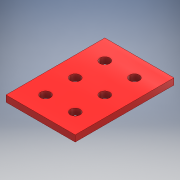
# Autodesk Inventor part: soportes celda de carga
Saved by Autodesk Inventor 2018 (Build 220112000, 112)
## iProperties
Created: 2019-05-18
Part Number: soportes celda de carga
Material: Generic
Document SubType Name: Modeling
Designer: JLVega003
Density: 1 g/cm^3
Appearance: Light Red
Author: JLVega003
Autodesk Inventor part; units mm, degrees
ref_plane "YZ Plane" through (0, 0, 0) normal (1, 0, 0) x (0, 1, 0)
ref_plane "XZ Plane" through (0, 0, 0) normal (0, 1, 0) x (-1, 0, 0)
ref_plane "XY Plane" through (0, 0, 0) normal (0, 0, 1) x (1, 0, 0)
sketch "Sketch1" plane through (0, 0, 0) normal (0, 0, 1) x (1, 0, 0)
  line L0 (17.5, -25) -> (-17.5, -25)
  line L1 (-17.5, -25) -> (-17.5, 25)
  line L2 (-17.5, 25) -> (17.5, 25)
  line L3 (17.5, 25) -> (17.5, -25)
  line L4 (17.5, -25) -> (-17.5, 25) construction
  line L5 (-17.5, -25) -> (17.5, 25) construction
  line L6 (7.5, -15) -> (-7.5, -15) construction
  line L7 (-7.5, -15) -> (-7.5, 15) construction
  line L8 (-7.5, 15) -> (7.5, 15) construction
  line L9 (7.5, 15) -> (7.5, -15) construction
  line L10 (7.5, -15) -> (-7.5, 15) construction
  line L11 (-7.5, -15) -> (7.5, 15) construction
  circle A0 centre (-7.5, 15) radius 2.5
  circle A1 centre (7.5, 15) radius 2.5
  circle A2 centre (-7.5, -15) radius 2.5
  circle A3 centre (7.5, -15) radius 2.5
  circle A4 centre (-7.5, 0) radius 2.5
  circle A5 centre (7.5, 0) radius 2.5
  point P0 (0, 0)
  dimension "d3" = 10
  dimension "d4" = 15
  dimension "d5" = 5
  dimension "d8" = 15
  dimension "d9" = 10
  constraints: 24 end point, 6 centre point, 6 midpoint, 5 equal radius, 4 coincident, 4 parallel, 2 horizontal, 2 perpendicular
  measures "d3" distance between parallel lines of L3 L9
  measures "d4" distance between parallel lines of L9 L7
  measures "d5" diameter of A0
  measures "d8" distance from line of A5.centre L8
  measures "d9" distance between parallel lines of L2 L8
extrude "Extrusion1" add sketch "Sketch1" along normal blind 3.175
body "Solid1"
